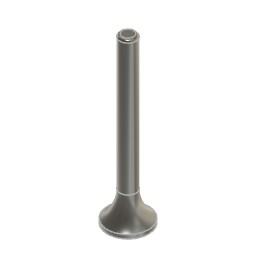
_5 inch 32mm pin.e6a95e00-5bcf-4c4b-87ae-00d59bb49d89 (Autodesk Fusion 360 design; units mm, degrees)
Autodesk Fusion 360 part; units mm, degrees
sketch "Sketch1" plane through (0, 0, 0) normal (1, 0, 0) x (0, 1, 0)
  line L0 (0, 0) -> (6.35, 0)
  line L1 (6.35, 0) -> (6.35, 125)
  line L2 (6.35, 125) -> (0, 125)
  line L3 (0, 125) -> (0, 0)
  line L4 (6.2544, 0) -> (6.2544, -3)
  line L5 (0, 0) -> (16, 0)
  arc A0 (6.35, 19.987) -> (16, 0) centre (31.8735, 19.987) ccw
  line L6 (0, 0) -> (16, 0)
  line L7 (16, 0) -> (16, -3)
  line L8 (16, -3) -> (0, -3)
  line L9 (0, -3) -> (0, 0)
  dimension "d1" = 6.35
  dimension "d2" = 125
  dimension "d5" = 16
  dimension "d6" = 3
  constraint horizontal L0
  constraint vertical L1
  constraint horizontal L2
  constraint vertical L3
  constraint coincident L0.start L3.end
  constraint vertical L4
  constraint perpendicular L3 L5
  constraint tangent L1 A0
  constraint coincident L1 A0.start
  constraint horizontal L6
  constraint vertical L7
  constraint horizontal L8
  constraint vertical L9
  measures "d1" distance of L0.start L0.end
  measures "d2" distance of L0.start L2.end
  measures "d5" distance of L0.start L5.end
  measures "d6" distance of L0.start L8.end
revolve "Revolve1" add sketch "Sketch1" angle 360 about axis through (0, 0, 125) along (0, 0, -1)
fillet "Fillet1" radius 2 1 edges at (-5.9203, 2.2963, 125)
